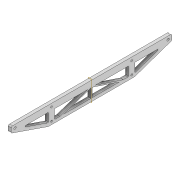
# Autodesk Inventor part: Horizontal_bar
Saved by Autodesk Inventor 2022 (Build 260153000, 153)
## iProperties
Created: 2022-08-23
Part Number: Horizontal_bar
Material: Generic
Document SubType Name: Modeling
Designer: dell
Density: 1 g/cm^3
Appearance: Default
Mass: 21.5376 g
Surface Area: 148.526 cm^2
Volume: 21.5376 cm^3
Author: dell
Autodesk Inventor part; units mm, degrees
ref_plane "YZ Plane" through (0, 0, 0) normal (1, 0, 0) x (0, 1, 0)
ref_plane "XZ Plane" through (0, 0, 0) normal (0, 1, 0) x (-1, 0, 0)
sketch "Sketch1" plane through (0, 0, 0) normal (1, 0, 0) x (0, 1, 0)
  line L0 (-5, 130) -> (-5, -130)
  line L1 (-5, -130) -> (5, -130)
  line L2 (5, -130) -> (5, 130)
  line L3 (5, 130) -> (-5, 130)
  line L4 (-5, 130) -> (5, -130) construction
  line L5 (-5, -130) -> (5, 130) construction
  circle A0 centre (0, -124) radius 1.95
  circle A1 centre (0, 124) radius 1.95
  line L6 (-5, -70) -> (-5, -60)
  circle A2 centre (0, -65) radius 1.5
  circle A3 centre (0, 65) radius 1.5
  point P0 (0, 0)
  point P1 (0, 0)
  dimension "d0" = 260
  dimension "d1" = 10
  dimension "d2" = 3.9
  dimension "d3" = 6
  dimension "d4" = 3.9
  dimension "d5" = 6
  dimension "d25" = 3
  dimension "d27" = 59
  dimension "d28" = 3
  dimension "d29" = 59
  constraints: 14 end point, 4 centre point, 3 midpoint, 2 parallel, 1 perpendicular, 1 point on line, 1 vertical, 1 vertical alignment
  measures "d0" distance of L0.start L0.end
  measures "d1" distance of L1.end L0.end
  measures "d2" diameter of A0
  measures "d3" distance from line of L1 A0.centre
  measures "d4" diameter of A1
  measures "d5" distance from line of L3 A1.centre
  measures "d25" diameter of A2
  measures "d27" distance of A0.centre A2.centre
  measures "d28" diameter of A3
  measures "d29" distance of A1.centre A3.centre
extrude "Extrusion1" add sketch "Sketch1" along normal blind 5
fillet "Fillet1" radius 2 4 edges at (2.5, 5, 130) (2.5, -5, 130) (2.5, 5, -130) (2.5, -5, -130)
sketch "Sketch2" plane through (5, 0, 0) normal (1, 0, 0) x (0, 0, -1)
  line L0 (-128, -5) -> (128, -5) projected
  line L1 (60, -5) -> (70, -5)
  line L2 (70, -5) -> (70, -25)
  line L3 (70, -25) -> (60, -25)
  line L4 (60, -25) -> (60, -5)
  circle A0 centre (65, -20) radius 1.5
  circle A1 centre (124, 0) radius 1.95 projected
  line L5 (70, -25) -> (128, -5)
  line L6 (70, -19.7111) -> (112.6621, -5)
  point P0 (0, 0)
  dimension "d15" = 3
  dimension "d16" = 20
  dimension "d17" = 5
  dimension "d18" = 10
  dimension "d20" = 59
  dimension "d23" = 5
  dimension "d32" = 5
  constraints: 12 end point, 3 parallel, 3 point on line, 1 centre point, 1 horizontal, 1 perpendicular
  measures "d15" diameter of A0
  measures "d16" vertical distance of point (0, 0) A0.centre
  measures "d17" distance from line of L3 A0.centre
  measures "d18" distance of L2.end L3.end
  measures "d20" horizontal distance of A0.centre A1.centre
  measures "d23" distance between parallel lines of L5 L6
  measures "d32" distance from line of L4 A0.centre
extrude "Extrusion2" add sketch "Sketch2" against normal blind 5 contours L0 L2 L3 L4 | L0 L5 L2 L6
mirror "Mirror1" about plane through (0, 0, 0) normal (0, 0, 1) of "Extrusion2"
sketch "Sketch4" plane through (5, 0, 0) normal (1, 0, 0) x (0, 0, -1)
  line L0 (-60, -25) -> (-60, -5) projected
  line L1 (60, -25) -> (60, -5) projected
  line L2 (-60, -25) -> (60, -25)
  line L3 (60, -25) -> (60, -20)
  line L4 (60, -20) -> (-60, -20)
  line L5 (-60, -20) -> (-60, -25)
  line L6 (-60, -25) -> (0, -5)
  line L7 (-60, -5) -> (60, -5) projected
  line L8 (70, -25) -> (60, -25) projected
  line L9 (0, -5) -> (60, -25)
  line L10 (60, -25) -> (60, -22.5)
  line L11 (6.3246, -5) -> (60, -22.8918)
  line L12 (-6.3246, -5) -> (-60, -22.8918)
  line L13 (-60, -5) -> (60, -5) projected
  line L14 (-1, -5) -> (1, -5)
  line L15 (1, -5) -> (1, -20)
  line L16 (1, -20) -> (-1, -20)
  line L17 (-1, -20) -> (-1, -5)
  point P0 (0, 0)
  point P1 (-60, -20)
  point P2 (-51.3246, -20)
  point P3 (-45, -20)
  point P4 (51.3246, -20)
  point P5 (45, -20)
  point P6 (-1, -5.3333)
  point P7 (-1, -20)
  point P8 (1, -5.3333)
  dimension "d33" = 5
  dimension "d37" = 2
  dimension "d38" = 2
  dimension "d39" = 1
  dimension "d40" = 1
  constraints: 26 end point, 7 point on line, 6 parallel, 2 horizontal, 2 midpoint, 2 perpendicular
  measures "d33" distance between parallel lines of L2 L4
  measures "d37" distance between parallel lines of L9 L11
  measures "d38" distance between parallel lines of L6 L12
  measures "d39" distance from line of point (0, 0) L15
  measures "d40" distance from line of point (0, 0) L17
extrude "Extrusion3" add sketch "Sketch4" against normal blind 5 contours L6 L4 L9 L2 | L0 L12 L4 L6 | L0 L4 L12 | L9 L4 L11 L1 | L4 L12 L7 L17 L6 | L11 L4 L1 | L9 L15 L7 L11 L4 | L17 L6 L9 L15 L4 | L17 L7 L6 | L9 L7 L15
fillet "Fillet3" radius 1 10 edges at (2.5, -19.7111, -70) (2.5, -5, -112.6621) (2.5, -5, -70) (2.5, -20, -60) (2.5, -5, -60) (2.5, -20, 60) (2.5, -5, 60) (2.5, -5, 112.6621) (2.5, -5, 70) (2.5, -19.7111, 70)
body "Solid1"
